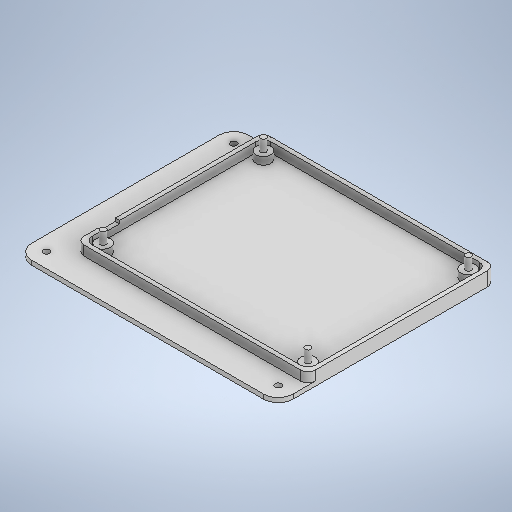
# Autodesk Inventor part: BottomCase
Saved by Autodesk Inventor 2025.2 (Build 292293000, 293)
## iProperties
Created: 2026-05-08
Part Number: BottomCase
Material: Generic
Document SubType Name: Modeling
Designer: Simon
Density: 1 g/cm^3
Appearance: Default
Author: Simon
Autodesk Inventor part; units mm, degrees
ref_plane "YZ Plane" through (0, 0, 0) normal (1, 0, 0) x (0, 1, 0)
ref_plane "XZ Plane" through (0, 0, 0) normal (0, 1, 0) x (-1, 0, 0)
ref_plane "XY Plane" through (0, 0, 0) normal (0, 0, 1) x (1, 0, 0)
sketch "Sketch1" plane through (0, 0, 0) normal (0, 1, 0) x (-1, 0, 0)
  line L0 (0, 0) -> (-176, 0)
  line L1 (-176, 0) -> (-176, -146)
  line L2 (-176, -146) -> (0, -146)
  line L3 (0, -146) -> (0, 0)
  line L4 (0, 0) -> (-176, 0)
  line L5 (-176, 0) -> (-176, -20)
  line L6 (-176, -20) -> (0, -20)
  line L7 (0, -20) -> (0, 0)
  line L8 (0, -146) -> (-20, -146)
  line L9 (-20, -146) -> (-20, 0)
  line L10 (-20, 0) -> (0, 0)
  line L11 (0, 0) -> (0, -146)
  line L12 (-20, -146) -> (-176, -146)
  line L13 (-176, -146) -> (-176, -143)
  line L14 (-176, -143) -> (-20, -143)
  line L15 (-20, -143) -> (-20, -146)
  line L16 (-20, -146) -> (-23, -146)
  line L17 (-23, -146) -> (-23, -20)
  line L18 (-23, -20) -> (-20, -20)
  line L19 (-20, -20) -> (-20, -146)
  line L20 (-20, -20) -> (-176, -20)
  line L21 (-176, -20) -> (-176, -23)
  line L22 (-176, -23) -> (-20, -23)
  line L23 (-20, -23) -> (-20, -20)
  line L24 (-176, -20) -> (-173, -20)
  line L25 (-173, -20) -> (-173, -146)
  line L26 (-173, -146) -> (-176, -146)
  line L27 (-176, -146) -> (-176, -20)
  line L28 (-20, -146) -> (-176, -146)
  line L29 (-176, -146) -> (-176, -143.2)
  line L30 (-176, -143.2) -> (-20, -143.2)
  line L31 (-20, -143.2) -> (-20, -146)
  line L32 (-176, -146) -> (-173.2, -146)
  line L33 (-173.2, -146) -> (-173.2, -20)
  line L34 (-173.2, -20) -> (-176, -20)
  line L35 (-176, -20) -> (-176, -146)
  line L36 (-176, -20) -> (-20, -20)
  line L37 (-20, -20) -> (-20, -22.8)
  line L38 (-20, -22.8) -> (-176, -22.8)
  line L39 (-176, -22.8) -> (-176, -20)
  line L40 (-20, -20) -> (-22.8, -20)
  line L41 (-22.8, -20) -> (-22.8, -146)
  line L42 (-22.8, -146) -> (-20, -146)
  line L43 (-20, -146) -> (-20, -20)
  line L44 (-23, -143) -> (-29, -143)
  line L45 (-29, -143) -> (-29, -137)
  line L46 (-29, -137) -> (-23, -137)
  line L47 (-23, -137) -> (-23, -143)
  line L48 (-173, -143) -> (-167, -143)
  line L49 (-167, -143) -> (-167, -137)
  line L50 (-167, -137) -> (-173, -137)
  line L51 (-173, -137) -> (-173, -143)
  line L52 (-173, -23) -> (-167, -23)
  line L53 (-167, -23) -> (-167, -29)
  line L54 (-167, -29) -> (-173, -29)
  line L55 (-173, -29) -> (-173, -23)
  line L56 (-23, -23) -> (-29, -23)
  line L57 (-29, -23) -> (-29, -29)
  line L58 (-29, -29) -> (-23, -29)
  line L59 (-23, -29) -> (-23, -23)
  line L60 (-23, -143) -> (-173, -143)
  line L61 (-173, -143) -> (-173, -23)
  line L62 (-173, -23) -> (-23, -23)
  line L63 (-23, -23) -> (-23, -143)
  circle A0 centre (-29, -137) radius 5
  circle A1 centre (-167, -137) radius 5
  circle A2 centre (-167, -29) radius 5
  circle A3 centre (-29, -29) radius 5
  line L64 (-22.8, -143.2) -> (-27.8, -143.2)
  line L65 (-27.8, -143.2) -> (-27.8, -138.2)
  line L66 (-27.8, -138.2) -> (-22.8, -138.2)
  line L67 (-22.8, -138.2) -> (-22.8, -143.2)
  line L68 (-173.2, -143.2) -> (-168.2, -143.2)
  line L69 (-168.2, -143.2) -> (-168.2, -138.2)
  line L70 (-168.2, -138.2) -> (-173.2, -138.2)
  line L71 (-173.2, -138.2) -> (-173.2, -143.2)
  line L72 (-173.2, -22.8) -> (-168.2, -22.8)
  line L73 (-168.2, -22.8) -> (-168.2, -27.8)
  line L74 (-168.2, -27.8) -> (-173.2, -27.8)
  line L75 (-173.2, -27.8) -> (-173.2, -22.8)
  line L76 (-22.8, -22.8) -> (-27.8, -22.8)
  line L77 (-27.8, -22.8) -> (-27.8, -27.8)
  line L78 (-27.8, -27.8) -> (-22.8, -27.8)
  line L79 (-22.8, -27.8) -> (-22.8, -22.8)
  circle A4 centre (-27.8, -138.2) radius 5
  circle A5 centre (-168.2, -138.2) radius 5
  circle A6 centre (-168.2, -27.8) radius 5
  circle A7 centre (-27.8, -27.8) radius 5
  dimension "d4" = 176
  dimension "d5" = 146
  dimension "d6" = 20
  dimension "d7" = 20
  dimension "d8" = 3
  dimension "d9" = 3
  dimension "d10" = 3
  dimension "d11" = 3
  dimension "d12" = 2.8
  dimension "d13" = 2.8
  dimension "d14" = 2.8
  dimension "d15" = 2.8
  dimension "d16" = 6
  dimension "d17" = 6
  dimension "d18" = 6
  dimension "d19" = 6
  dimension "d20" = 6
  dimension "d21" = 6
  dimension "d22" = 6
  dimension "d23" = 6
  dimension "d24" = 10
  dimension "d25" = 10
  dimension "d26" = 10
  dimension "d27" = 10
  dimension "d28" = 5
  dimension "d29" = 5
  dimension "d30" = 5
  dimension "d31" = 5
  dimension "d32" = 5
  dimension "d33" = 5
  dimension "d34" = 5
  dimension "d35" = 5
  constraints: 160 end point, 40 parallel, 26 point on line, 20 horizontal, 20 perpendicular, 8 coincident, 4 centre point, 2 horizontal alignment, 2 vertical alignment, 8 other
  measures "d4" distance of L2.end L1.end
  measures "d5" distance of L1.end L0.end
  measures "d6" distance of L5.end L4.end
  measures "d7" distance of L9.end L10.end
  measures "d8" distance of L12.end L13.end
  measures "d9" distance of L17.end L18.end
  measures "d10" distance of L21.end L20.end
  measures "d11" distance of L25.end L26.end
  measures "d12" distance of L28.end L29.end
  measures "d13" distance of L34.end L33.end
  measures "d14" distance of L36.end L37.end
  measures "d15" distance of L42.end L41.end
  measures "d16" distance of L45.end L46.end
  measures "d17" distance of L44.end L45.end
  measures "d18" distance of L50.end L49.end
  measures "d19" distance of L49.end L48.end
  measures "d20" distance of L53.end L54.end
  measures "d21" distance of L52.end L53.end
  measures "d22" distance of L58.end L57.end
  measures "d23" distance of L57.end L56.end
  measures "d24" diameter of A0
  measures "d25" diameter of A1
  measures "d26" diameter of A2
  measures "d27" diameter of A3
  measures "d28" distance of L65.end L66.end
  measures "d29" distance of L64.end L65.end
  measures "d30" distance of L70.end L69.end
  measures "d31" distance of L69.end L68.end
  measures "d32" distance of L73.end L74.end
  measures "d33" distance of L72.end L73.end
  measures "d34" distance of L78.end L77.end
  measures "d35" distance of L77.end L76.end
extrude "Extrusion1" add sketch "Sketch1" against normal blind 3
extrude "Extrusion2" add sketch "Sketch1" along normal blind 5 contours L77 L78 A3 L58 L57 | A3 L78 L77 | A7 A3 | A3 L57 L58 A7 | L74 L73 A2 L53 L54 | A2 L73 L74 | A6 A2 | A2 L54 L53 A6 | L66 L65 A0 L45 L46 | A0 L65 L66 | A4 A0 | A0 L46 L45 A4 | L70 L69 A1 | A1 L50 L49 L69 L70 | A5 A1 L49 L50 | A1 A5
extrude "Extrusion4" add sketch "Sketch1" along normal blind 6.5 contours L9 L38 L41 L6 | L6 L33 L38 L1 | L41 L38 L17 L6 | L9 L22 L41 L38 | L2 L41 L30 L9 | L38 L33 L22 L1 | L6 L25 L38 L33 | L17 L38 L25 L6 | L9 L14 L41 L22 | L2 L17 L30 L41 | L30 L41 L14 L9 | L22 L33 L14 L1 | L2 L25 L30 L17 | L14 L33 L30 L1 | L2 L33 L30 L25 | L30 L33 L2 L1
fillet "Fillet1" radius 5 4 edges at (22.8, 3.25, -143.2) (22.8, 3.25, -22.8) (173.2, 3.25, -22.8) (173.2, 3.25, -143.2)
sketch "Sketch2" plane through (29, 5, -137) normal (0, 1, 0) x (1, 0, 0)
  circle A0 centre (0, 0) radius 1.95
  circle A1 centre (138, 0) radius 5 projected
  circle A2 centre (138, 0) radius 1.95
  circle A3 centre (138, -108) radius 5 projected
  circle A4 centre (138, -108) radius 1.95
  circle A5 centre (0, -108) radius 5 projected
  circle A6 centre (0, -108) radius 1.95
  point P0 (-29, -137)
  dimension "d45" = 3.9
  dimension "d46" = 3.9
  dimension "d47" = 3.9
  dimension "d48" = 3.9
  constraints: 4 centre point, 3 coincident
  measures "d45" diameter of A0
  measures "d46" diameter of A2
  measures "d47" diameter of A4
  measures "d48" diameter of A6
extrude "Extrusion5" add sketch "Sketch2" along normal blind 8 contours A0 | A2 | A4 | A6
fillet "Fillet2" radius 5 4 edges at (176, 3.25, -20) (20, 3.25, -20) (176, 1.75, -146) (20, 3.25, -146)
fillet "Fillet3" radius 10 3 edges at (176, -1.5, 0) (0, -1.5, 0) (0, -1.5, -146)
sketch "Sketch3" plane through (0, 0, 0) normal (0, 1, 0) x (1, 0, 0)
  line L0 (25, 146) -> (10, 146) projected
  line L1 (0, 0) -> (20, 0)
  line L2 (20, 0) -> (20, 146)
  line L3 (20, 146) -> (0, 146)
  line L4 (0, 146) -> (0, 0)
  line L5 (176, 10) -> (176, 25) projected
  line L6 (0, 0) -> (176, 0)
  line L7 (176, 0) -> (176, 20)
  line L8 (176, 20) -> (0, 20)
  line L9 (0, 20) -> (0, 0)
  line L10 (20, 20) -> (0, 0)
  line L11 (20, 0) -> (0, 20)
  line L12 (176, 0) -> (156, 0)
  line L13 (156, 0) -> (156, 20)
  line L14 (156, 20) -> (176, 20)
  line L15 (176, 20) -> (176, 0)
  line L16 (0, 146) -> (20, 146)
  line L17 (20, 146) -> (20, 126)
  line L18 (20, 126) -> (0, 126)
  line L19 (0, 126) -> (0, 146)
  line L20 (20, 126) -> (0, 146)
  line L21 (20, 146) -> (0, 126)
  line L22 (176, 0) -> (156, 20)
  line L23 (156, 0) -> (176, 20)
  line L24 (166, 10) -> (10, 10)
  line L25 (10, 136) -> (10, 10)
  circle A0 centre (10, 136) radius 2.15
  circle A1 centre (10, 10) radius 2.15
  circle A2 centre (166, 10) radius 2.15
  dimension "d53" = 20
  dimension "d54" = 20
  dimension "d55" = 20
  dimension "d56" = 20
  dimension "d57" = 4.3
  dimension "d58" = 4.3
  dimension "d59" = 4.3
  constraints: 48 end point, 8 parallel, 6 point on line, 5 perpendicular, 4 horizontal, 3 centre point, 3 coincident, 3 midpoint
  measures "d53" distance of L3.end L2.end
  measures "d54" distance of L7.end L6.end
  measures "d55" distance of L13.end L14.end
  measures "d56" distance of L16.end L17.end
  measures "d57" diameter of A0
  measures "d58" diameter of A1
  measures "d59" diameter of A2
extrude "Extrusion6" cut sketch "Sketch3" against normal blind 8 contours A0 L20 L21 | L21 L20 A0 | A0 L25 L20 | L21 A0 L20 | L25 A0 L21 | A1 L24 L10 | L10 L25 A1 | A1 L11 L24 | A2 L23 L22 | L22 L24 A2 | L25 L11 A1 | L11 A1 L10 | L10 A1 L11 | L24 L23 A2 | A2 L22 L23 | L22 A2 L23
sketch "Sketch4" plane through (0, 6.5, 0) normal (0, 1, 0) x (1, 0, 0)
  arc A0 (20, 25) -> (25, 20) centre (25, 25) ccw projected
  line L0 (25, 20) -> (20, 20)
  line L1 (20, 20) -> (20, 25)
  line L2 (20, 25) -> (25, 25)
  line L3 (25, 25) -> (25, 20)
  line L4 (22.8, 27.8) -> (22.8, 138.2) projected
  line L5 (20, 20) -> (22.8, 20)
  line L6 (22.8, 20) -> (22.8, 34.25)
  line L7 (22.8, 34.25) -> (20, 34.25)
  line L8 (20, 34.25) -> (20, 20)
  line L9 (20, 34.25) -> (22.8, 34.25)
  line L10 (22.8, 34.25) -> (22.8, 46.25)
  line L11 (22.8, 46.25) -> (20, 46.25)
  line L12 (20, 46.25) -> (20, 34.25)
  point P0 (0, 0)
  dimension "d62" = 14.25
  dimension "d63" = 12
  constraints: 24 end point, 6 parallel, 3 horizontal, 3 perpendicular, 2 point on line
  measures "d62" distance of L6.end L5.end
  measures "d63" distance of L10.end L9.end
extrude "Extrusion7" cut sketch "Sketch4" against normal blind 2 contours L12 L11 L4 L7
body "Solid1"
